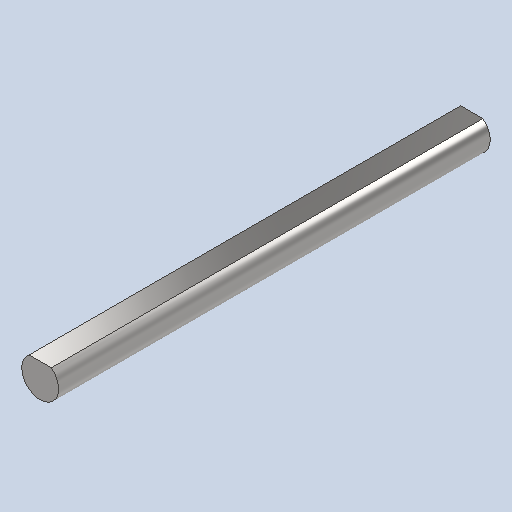
# Autodesk Inventor part: ServoShaft
Saved by Autodesk Inventor 2023 (Build 270158000, 158)
## iProperties
Created: 2021-01-26
Part Number: ServoShaft
Material: Stainless Steel
Document SubType Name: Modeling
Designer: valer
Density: 8 g/cm^3
Appearance: Semi-Polished
Author: valer
Autodesk Inventor part; units mm, degrees
ref_plane "YZ Plane" through (0, 0, 0) normal (1, 0, 0) x (0, 1, 0)
ref_plane "XZ Plane" through (0, 0, 0) normal (0, 1, 0) x (-1, 0, 0)
ref_plane "XY Plane" through (0, 0, 0) normal (0, 0, 1) x (1, 0, 0)
sketch "Sketch1" plane through (0, 0, 0) normal (0, 0, 1) x (1, 0, 0)
  circle A0 centre (0, 0) radius 3
  line L0 (0, 0) -> (0, -3) construction
  line L1 (-1.8, 2.4) -> (1.8, 2.4)
  dimension "d0" = 6
  dimension "d1" = 5.4
  constraints: 4 end point, 3 point on circle, 1 centre point, 1 coincident, 1 horizontal, 1 vertical
  measures "d0" diameter of A0
  measures "d1" distance from line of L0.end L1
extrude "Extrusion1" add sketch "Sketch1" along normal blind 70 contours A0 L1 picked at (0.3021, 0.4498)
body "Solid1"
